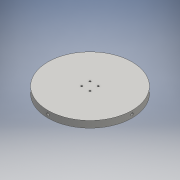
# Autodesk Inventor part: outsideBottom2
Saved by Autodesk Inventor 2016 (Build 200138000, 138)
## iProperties
Created: 2016-11-12
Part Number: outsideBottom2
Material: 一般
Document SubType Name: Modeling
Designer: Daisuke
Density: 1 g/cm^3
Appearance: 既定
Author: Daisuke
Autodesk Inventor part; units mm, degrees
sketch "スケッチ1" plane through (0, 0, 0) normal (0, 0, 1) x (1, 0, 0)
  circle A0 centre (0, 0) radius 50.5
  dimension "d0" = 101
  constraints: 1 centre point, 1 coincident
  measures "d0" diameter of A0
extrude "押し出し1" add sketch "スケッチ1" along normal blind 8
sketch "スケッチ2" plane through (0, 0, 8) normal (0, 0, 1) x (1, 0, 0)
  line L0 (-5, -5) -> (5, -5) construction
  line L1 (5, -5) -> (5, 5) construction
  line L2 (5, 5) -> (-5, 5) construction
  line L3 (-5, 5) -> (-5, -5) construction
  line L4 (-5, -5) -> (5, 5) construction
  line L5 (5, -5) -> (-5, 5) construction
  circle A0 centre (-5, 5) radius 1
  circle A1 centre (5, 5) radius 1
  circle A2 centre (5, -5) radius 1
  circle A3 centre (-5, -5) radius 1
  point P0 (0, 0)
  dimension "d3" = 10
  dimension "d4" = 10
  dimension "d5" = 2
  dimension "d6" = 2
  dimension "d7" = 2
  dimension "d8" = 2
  constraints: 12 end point, 4 centre point, 4 coincident, 2 midpoint, 2 parallel, 1 horizontal, 1 perpendicular
  measures "d3" distance of L2.end L1.end
  measures "d4" distance of L1.end L0.end
  measures "d5" diameter of A0
  measures "d6" diameter of A1
  measures "d7" diameter of A2
  measures "d8" diameter of A3
extrude "押し出し2" cut sketch "スケッチ2" against normal blind 8
ref_plane "作業平面1" through (50.5, 0, 0) normal (1, 0, 0) x (0, 1, 0)
ref_plane "作業平面2" through (-50.5, 0, 0) normal (1, 0, 0) x (0, 1, 0)
ref_plane "作業平面3" through (0, 50.5, 0) normal (0, 1, 0) x (-1, 0, 0)
ref_plane "作業平面4" through (0, -50.5, 0) normal (0, 1, 0) x (-1, 0, 0)
sketch "スケッチ3" plane through (50.5, 0, 0) normal (1, 0, 0) x (0, 1, 0)
  line L0 (0, 0) -> (0, 4) construction
  circle A0 centre (0, 4) radius 1.5
  dimension "d14" = 4
  dimension "d15" = 3
  constraints: 2 end point, 1 centre point, 1 coincident, 1 vertical
  measures "d14" distance of L0.start L0.end
  measures "d15" diameter of A0
extrude "押し出し3" cut sketch "スケッチ3" against normal blind 5
sketch "スケッチ4" plane through (-50.5, 0, 0) normal (1, 0, 0) x (0, 1, 0)
  line L0 (0, 0) -> (0, 4) construction
  circle A0 centre (0, 4) radius 1.5
  dimension "d18" = 4
  dimension "d19" = 3
  constraints: 2 end point, 1 centre point, 1 coincident, 1 vertical
  measures "d18" distance of L0.start L0.end
  measures "d19" diameter of A0
extrude "押し出し4" cut sketch "スケッチ4" along normal blind 5
sketch "スケッチ5" plane through (0, 50.5, 0) normal (0, 1, 0) x (-1, 0, 0)
  line L0 (0, 0) -> (0, 4) construction
  circle A0 centre (0, 4) radius 1.5
  dimension "d22" = 4
  dimension "d23" = 3
  constraints: 2 end point, 1 centre point, 1 coincident, 1 vertical
  measures "d22" distance of L0.start L0.end
  measures "d23" diameter of A0
extrude "押し出し5" cut sketch "スケッチ5" against normal blind 5
sketch "スケッチ6" plane through (0, -50.5, 0) normal (0, 1, 0) x (-1, 0, 0)
  line L0 (0, 0) -> (0, 4) construction
  circle A0 centre (0, 4) radius 1.5
  dimension "d26" = 4
  dimension "d27" = 3
  constraints: 2 end point, 1 centre point, 1 coincident, 1 vertical
  measures "d26" distance of L0.start L0.end
  measures "d27" diameter of A0
extrude "押し出し6" cut sketch "スケッチ6" along normal blind 5
thread "ねじ1" size "M3x0.5" class "6H" standard "ANSI Metric M Profile" full length
thread "ねじ2" size "M3x0.5" class "6H" standard "ANSI Metric M Profile" full length
thread "ねじ3" size "M3x0.5" class "6H" standard "ANSI Metric M Profile" full length
thread "ねじ4" size "M3x0.5" class "6H" standard "ANSI Metric M Profile" full length
thread "ねじ5" size "M2x0.4" class "6H" standard "ANSI Metric M Profile" full length
thread "ねじ6" size "M2x0.4" class "6H" standard "ANSI Metric M Profile" full length
thread "ねじ7" size "M2x0.4" class "6H" standard "ANSI Metric M Profile" full length
thread "ねじ8" size "M2x0.4" class "6H" standard "ANSI Metric M Profile" full length
